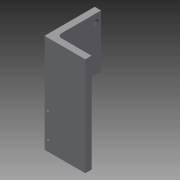
# Autodesk Inventor part: Left Angle
Saved by Autodesk Inventor 2013 (Build 170138000, 138)
## iProperties
Created: 2012-09-25
Part Number: Left Angle
Material: Generic
Document SubType Name: Modeling
Designer: uqgtayle
Density: 1 g/cm^3
Author: uqgtayle
Autodesk Inventor part; units mm, degrees
ref_plane "YZ Plane" through (0, 0, 0) normal (1, 0, 0) x (0, 1, 0)
ref_plane "XZ Plane" through (0, 0, 0) normal (0, 1, 0) x (-1, 0, 0)
ref_plane "XY Plane" through (0, 0, 0) normal (0, 0, 1) x (1, 0, 0)
sketch "Sketch1" plane through (0, 0, 0) normal (0, 0, 1) x (1, 0, 0)
  line L0 (0, 38.2) -> (0, 0)
  line L1 (0, 0) -> (31, 0)
  line L2 (31, 0) -> (31, 4.8)
  line L3 (31, 4.8) -> (7.8, 4.8)
  line L4 (4.8, 7.8) -> (4.8, 38.2)
  line L5 (4.8, 38.2) -> (0, 38.2)
  arc A0 (4.8, 7.8) -> (7.8, 4.8) centre (7.8, 7.8) ccw
  dimension "d0" = 31
  dimension "d1" = 38.2
  dimension "d2" = 4.8
  dimension "d3" = 4.8
  dimension "d4" = 3
  constraints: 12 end point, 4 parallel, 2 point on circle, 2 tangent, 1 centre point, 1 perpendicular, 1 vertical
  measures "d0" distance of L1.end L0.end
  measures "d1" distance of L0.start L0.end
  measures "d2" distance of L1.end L2.end
  measures "d3" distance of L0.start L4.end
  measures "d4" radius of A0
extrude "Extrusion1" add sketch "Sketch1" against normal blind 75
sketch "Sketch2" plane through (0, 0, 0) normal (-1, 0, 0) x (0, 0, 1)
  line L0 (0, 0) -> (0, 38.2) projected
  line L1 (0, 38.2) -> (-75, 38.2) projected
  point P0 (-6, 34.2)
  dimension "d7" = 4
  dimension "d8" = 6
  measures "d7" distance from line of L1 point (-6, 34.2)
  measures "d8" distance from line of point (-6, 34.2) L0
hole "Hole1" at (0, 34.2, -6) direction (1, 0, 0) diameter 4.134 end through all thread size "M5x0.8" class "6H" standard "ANSI Metric M Profile"
sketch "Sketch3" plane through (0, 0, 0) normal (-1, 0, 0) x (0, 0, 1)
  line L0 (0, 0) -> (0, 38.2) projected
  line L1 (0, 38.2) -> (-75, 38.2) projected
  line L2 (-100.4339, 50.496) -> (-40, 50.496)
  line L3 (-40, 50.496) -> (-40, 28.2)
  line L4 (-40, 28.2) -> (-100.4339, 28.2)
  line L5 (-100.4339, 28.2) -> (-100.4339, 50.496)
  dimension "d16" = 40
  dimension "d17" = 10
  constraints: 8 end point, 2 parallel, 1 horizontal, 1 perpendicular
  measures "d16" distance between parallel lines of L3 L0
  measures "d17" distance between parallel lines of L4 L1
extrude "Extrusion2" cut sketch "Sketch3" against normal through all
sketch "Sketch4" plane through (0, 28.2, -40) normal (0, 1, 0) x (1, 0, 0)
  line L0 (0, 35) -> (4.8, 35) projected
  line L1 (0, 0) -> (4.8, 0) projected
  point P0 (0, -40)
  point P1 (2.4, 27)
  point P2 (2.4, 8)
  dimension "d20" = 8
  dimension "d21" = 8
  dimension "d22" = 19
  measures "d20" distance from line of point (2.4, 8) L1
  measures "d21" distance from line of point (2.4, 27) L0
  measures "d22" distance of point (2.4, 8) point (2.4, 27)
hole "Hole2" at (2.4, 28.2, -67) at (2.4, 28.2, -48) direction (0, -1, 0) diameter 1.567 end through all thread size "M2x0.4" class "6H" standard "ISO Metric profile"
body "Solid1"
